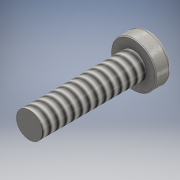
# Autodesk Inventor part: plastic_screw_3_x_12
Saved by Autodesk Inventor 2016 (Build 200138000, 138)
## iProperties
Created: 2016-11-04
Part Number: plastic_screw_3_x_12
Material: Generic
Document SubType Name: Modeling
Designer: hesaon
Density: 1 g/cm^3
Appearance: Default
Author: hesaon
Autodesk Inventor part; units mm, degrees
ref_plane "YZ Plane" through (0, 0, 0) normal (1, 0, 0) x (0, 1, 0)
ref_plane "XZ Plane" through (0, 0, 0) normal (0, 1, 0) x (-1, 0, 0)
ref_plane "XY Plane" through (0, 0, 0) normal (0, 0, 1) x (1, 0, 0)
sketch "Sketch1" plane through (0, 0, 0) normal (0, 1, 0) x (-1, 0, 0)
  circle A0 centre (0, 0) radius 1.5
  dimension "d0" = 3
  constraints: 1 centre point, 1 coincident
  measures "d0" diameter of A0
extrude "Extrusion1" add sketch "Sketch1" along normal blind 12
sketch "Sketch2" plane through (0, 12, 0) normal (0, 1, 0) x (1, 0, 0)
  circle A0 centre (0, 0) radius 2.6
  dimension "d3" = 5.2
  constraints: 1 centre point, 1 coincident
  measures "d3" diameter of A0
extrude "Extrusion2" add sketch "Sketch2" along normal blind 2
sketch "Sketch3" plane through (0, 14, 0) normal (0, 1, 0) x (1, 0, 0)
  line L0 (-1.8, 0.5) -> (-0.8, 0.5)
  line L1 (-0.8, 0.5) -> (-0.5, 0.8)
  line L2 (-0.5, 0.8) -> (-0.5, 1.8)
  line L3 (-0.5, 1.8) -> (0.5, 1.8)
  line L4 (0.5, 1.8) -> (0.5, 0.8)
  line L5 (0.5, 0.8) -> (0.8, 0.5)
  line L6 (0.8, 0.5) -> (1.8, 0.5)
  line L7 (1.8, 0.5) -> (1.8, -0.5)
  line L8 (1.8, -0.5) -> (0.8, -0.5)
  line L9 (0.8, -0.5) -> (0.5, -0.8)
  line L10 (0.5, -0.8) -> (0.5, -1.8)
  line L11 (0.5, -1.8) -> (-0.5, -1.8)
  line L12 (-0.5, -1.8) -> (-0.5, -0.8)
  line L13 (-0.5, -0.8) -> (-0.8, -0.5)
  line L14 (-0.8, -0.5) -> (-1.8, -0.5)
  line L15 (-1.8, -0.5) -> (-1.8, 0.5)
  point P0 (0, 0)
  dimension "d6" = 1
  dimension "d7" = 1
  dimension "d8" = 1
  dimension "d9" = 1
  dimension "d11" = 1
  dimension "d12" = 1
  dimension "d13" = 1
  dimension "d14" = 1
  dimension "d15" = 1
  dimension "d16" = 1
  dimension "d17" = 135
  dimension "d18" = 135
  dimension "d19" = 135
  dimension "d20" = 0.5
  dimension "d21" = 0.5
  dimension "d22" = 1.8
  dimension "d23" = 1.8
  dimension "d24" = 0.5
  constraints: 32 end point, 7 perpendicular, 4 point on line, 2 equal length, 1 vertical
  measures "d6" distance of L14.end L0.start
  measures "d7" distance of L3.end L2.end
  measures "d8" distance of L6.end L7.end
  measures "d9" distance of L0.end L0.start
  measures "d11" distance of L11.end L12.end
  measures "d12" distance of L9.end L10.end
  measures "d13" distance of L7.end L8.end
  measures "d14" distance of L5.end L6.end
  measures "d15" distance of L3.end L4.end
  measures "d16" distance of L2.end L1.end
  measures "d17" angle of L0 L1
  measures "d18" angle of L4 L5
  measures "d19" angle of L10 L9
  measures "d20" distance from line of point (0, 0) L14
  measures "d21" horizontal distance of point (0, 0) L11.end
  measures "d22" distance from line of point (0, 0) L7
  measures "d23" distance from line of point (0, 0) L15
  measures "d24" distance from line of point (0, 0) L2
extrude "Extrusion3" cut sketch "Sketch3" against normal blind 0.8
fillet "Fillet1" radius 0.5 1 edges at (-2.6, 14, 0)
fillet "Fillet2" radius 0.1 1 edges at (-2.6, 12, 0)
thread "Thread1" size "G 1/16-28" class "A" standard "BSP Pipe Threads" full length
equation "\"d7\" = d6"
equation "\"d8\" = d6"
equation "\"d9\" = d6"
equation "\"d11\" = d6"
equation "\"d12\" = d6"
equation "\"d13\" = d6"
equation "\"d14\" = d6"
equation "\"d15\" = d6"
equation "\"d16\" = d6"
equation "\"d18\" = d17"
equation "\"d19\" = d17"
equation "\"d20\" = 0.5 * d16"
equation "\"d21\" = 0.5 * d16"
equation "\"d24\" = 0.5 * d16"
body "Solid1"
